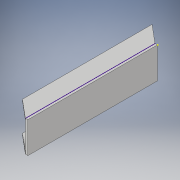
# Autodesk Inventor part: elevation
Saved by Autodesk Inventor 2019 (Build 230136000, 136)
## iProperties
Created: 2020-03-04
Part Number: elevation
Material: Generic
Document SubType Name: Modeling
Designer: Lenovo
Density: 1 g/cm^3
Appearance: Default
Author: Lenovo
Autodesk Inventor part; units mm, degrees
ref_plane "YZ Plane" through (0, 0, 0) normal (1, 0, 0) x (0, 1, 0)
ref_plane "XZ Plane" through (0, 0, 0) normal (0, 1, 0) x (-1, 0, 0)
ref_plane "XY Plane" through (0, 0, 0) normal (0, 0, 1) x (1, 0, 0)
sketch "Sketch1" plane through (0, 0, 0) normal (1, 0, 0) x (0, 1, 0)
  line L0 (0, 0) -> (-60, 0)
  line L1 (-60, 0) -> (-60, 250)
  line L2 (-60, 250) -> (0, 250)
  line L3 (0, 250) -> (0, 0)
  dimension "d0" = 60
  dimension "d1" = 250
  constraints: 8 end point, 2 parallel, 1 horizontal, 1 perpendicular
  measures "d0" distance of L1.end L2.end
  measures "d1" distance of L0.end L1.end
extrude "Extrusion1" add sketch "Sketch1" along normal blind 5
sketch "Sketch2" plane through (5, 0, 0) normal (1, 0, 0) x (0, 0, -1)
  point P0 (0, 0)
sketch "Sketch3" plane through (0, 0, 250) normal (0, 1, 0) x (1, 0, 0)
  line L0 (-34.5249, 250) -> (-35, 250)
  line L1 (0, 250) -> (-34.5249, 278.9698)
  line L2 (0, 250) -> (45.069, 250) construction
  line L3 (-34.5249, 0) -> (-35, 0)
  line L4 (0, 0) -> (-34.5249, 28.9698)
  line L5 (0, 0) -> (45.069, 0) construction
  line L6 (-34.5249, 28.9698) -> (-34.5249, 278.9698)
  line L7 (0, 0) -> (0, 250)
  dimension "d4" = 35
  dimension "d5" = 45.069
  dimension "d6" = 140
  dimension "d7" = 35
  dimension "d8" = 45.069
  dimension "d9" = 140
  constraints: 16 end point, 4 horizontal, 2 equal length, 2 point on line, 1 vertical
  measures "d4" distance of L1.start L0.end
  measures "d5" distance of L1.start L1.end
  measures "d6" angle of L2 L1
  measures "d7" distance of L4.start L3.end
  measures "d8" distance of L4.start L4.end
  measures "d9" angle of L5 L4
sketch "Sketch4" plane through (0, 0, 250) normal (0, 1, 0) x (1, 0, 0)
  line L0 (0, 0) -> (0, 250)
  constraints: 2 end point, 1 vertical
extrude "Extrusion2" add sketch "Sketch3" against normal blind 3
sketch "Sketch5" plane through (0, -60, 0) normal (0, -1, 0) x (1, 0, 0)
  line L0 (0, 0) -> (-34.5249, -28.9698)
  line L1 (-34.5249, -28.9698) -> (-34.5249, 221.0302)
  line L2 (-34.5249, 221.0302) -> (0, 250)
  line L3 (0, 250) -> (0, 0)
  constraints: 8 end point, 2 parallel, 1 vertical
extrude "Extrusion3" add sketch "Sketch5" against normal blind 3
body "Solid1"
